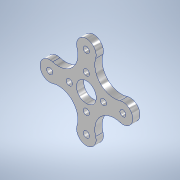
# Autodesk Inventor part: 関節1_プーリ接続
Saved by Autodesk Inventor 2021 (Build 250183000, 183)
## iProperties
Created: 2022-02-02
Part Number: 関節1_プーリ接続
Material: アルミニウム 6061
Document SubType Name: Modeling
Designer: hirohumi
Density: 2.7 g/cm^3
Appearance: アルミニウム - フラット
Author: hirohumi
Autodesk Inventor part; units mm, degrees
ref_plane "YZ Plane" through (0, 0, 0) normal (1, 0, 0) x (0, 1, 0)
ref_plane "XZ Plane" through (0, 0, 0) normal (0, 1, 0) x (-1, 0, 0)
ref_plane "XY Plane" through (0, 0, 0) normal (0, 0, 1) x (1, 0, 0)
sketch "スケッチ1" plane through (0, 0, 0) normal (0, 0, 1) x (1, 0, 0)
  circle A0 centre (0, 0) radius 4.05
  circle A1 centre (0, 0) radius 15 construction
  circle A2 centre (0, 0) radius 7 construction
  circle A3 centre (0, 15) radius 1.25
  circle A4 centre (0, 7) radius 1.25
  circle A5 centre (-15, 0) radius 1.25
  circle A6 centre (-7, 0) radius 1.25
  circle A7 centre (0, -15) radius 1.25
  circle A8 centre (0, -7) radius 1.25
  circle A9 centre (15, 0) radius 1.25
  circle A10 centre (7, 0) radius 1.25
  arc A11 (3.8229, 13.8229) -> (-3.8229, 13.8229) centre (0, 15) ccw
  arc A12 (-13.8229, 3.8229) -> (-13.8229, -3.8229) centre (-15, 0) ccw
  arc A13 (-3.8229, -13.8229) -> (3.8229, -13.8229) centre (0, -15) ccw
  arc A14 (13.8229, -3.8229) -> (13.8229, 3.8229) centre (15, 0) ccw
  arc A15 (-13.8229, 3.8229) -> (-3.8229, 13.8229) centre (-11.4686, 11.4686) ccw
  arc A16 (3.8229, 13.8229) -> (13.8229, 3.8229) centre (11.4686, 11.4686) ccw
  arc A17 (-3.8229, -13.8229) -> (-13.8229, -3.8229) centre (-11.4686, -11.4686) ccw
  arc A18 (13.8229, -3.8229) -> (3.8229, -13.8229) centre (11.4686, -11.4686) ccw
  dimension "d2" = 14
  dimension "d0" = 8.1
  dimension "d1" = 30
  dimension "d3" = 2.5
  dimension "d4" = 2.5
  dimension "d7" = 360
  dimension "d9" = 4
  dimension "d10" = 4
  dimension "d11" = 4
  dimension "d12" = 4
  dimension "d13" = 8
  dimension "d14" = 8
  dimension "d15" = 8
  dimension "d16" = 8
  constraints: 18 centre point, 18 point on circle, 8 tangent, 7 coincident, 3 vertical alignment, 19 other
  measures "d0" diameter of A0
  measures "d1" diameter of A1
  measures "d3" diameter of A3
  measures "d4" diameter of A4
  measures "d9" radius of A14
  measures "d10" radius of A11
  measures "d11" radius of A12
  measures "d12" radius of A13
  measures "d13" radius of A15
  measures "d14" radius of A17
  measures "d15" radius of A18
  measures "d16" radius of A16
extrude "押し出し1" add sketch "スケッチ1" along normal blind 3
